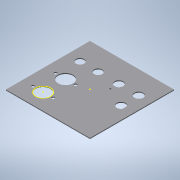
# Autodesk Inventor part: AmplifierPowerSupplyNew
Saved by Autodesk Inventor 2020 (Build 240168000, 168)
## iProperties
Created: 2013-08-12
Part Number: AmplifierPowerSupplyNew
Material: Generic
Document SubType Name: Modeling
Designer: laird
Density: 1 g/cm^3
Appearance: Default
Mass: 14.4778 g
Surface Area: 298.659 cm^2
Volume: 14.4778 cm^3
Author: laird
Title: Top plate
Autodesk Inventor part; units mm, degrees
ref_plane "YZ Plane" through (0, 0, 0) normal (1, 0, 0) x (0, 1, 0)
ref_plane "XZ Plane" through (0, 0, 0) normal (0, 1, 0) x (-1, 0, 0)
ref_plane "XY Plane" through (0, 0, 0) normal (0, 0, 1) x (1, 0, 0)
sketch "Sketch1" plane through (0, 0, 0) normal (0, 0, 1) x (1, 0, 0)
  line L0 (0, 46.5) -> (46.5, 46.5)
  line L1 (46.5, 46.5) -> (46.5, 0)
  line L2 (46.5, 0) -> (46.5, -46.5)
  line L3 (46.5, -46.5) -> (0, -46.5)
  line L4 (0, -46.5) -> (-46.5, -46.5)
  line L5 (-46.5, -46.5) -> (-46.5, 0)
  line L6 (-46.5, 0) -> (-46.5, 46.5)
  line L7 (-46.5, 46.5) -> (0, 46.5)
  point P0 (0, 0)
  dimension "d82" = 46.5
  dimension "d83" = 46.5
  dimension "d84" = 93
  dimension "d85" = 93
  constraints: 16 end point, 4 perpendicular, 4 point on line, 1 horizontal
  measures "d82" distance of L1.end L2.end
  measures "d83" distance of L3.end L4.end
  measures "d84" distance of L0.end L6.end
  measures "d85" distance of L2.end L0.end
extrude "Plate" add sketch "Sketch1" along normal blind 1
sketch "Sketch2" plane through (0, 0, 1) normal (0, 0, 1) x (1, 0, 0)
  circle A0 centre (-23.5, -28.5) radius 8.25
  circle A1 centre (-12.4, -28.5) radius 1.7
  circle A2 centre (-34.6, -28.5) radius 1.7
  line L0 (-46.5, 46.5) -> (-46.5, -46.5) projected
  line L1 (-46.5, -46.5) -> (46.5, -46.5) projected
  point P0 (0, 0)
  dimension "d6" = 16.5
  dimension "d8" = 3.4
  dimension "d29" = 11.1
  dimension "d30" = 11.1
  dimension "d93" = 23
  dimension "d94" = 18
  constraints: 3 centre point, 1 equal radius
  measures "d6" diameter of A0
  measures "d8" diameter of A2
  measures "d29" distance of A0.centre A1.centre
  measures "d30" distance of A0.centre A2.centre
  measures "d93" distance from line of L0 A0.centre
  measures "d94" distance from line of L1 A0.centre
extrude "DIN hole" cut sketch "Sketch2" against normal through all
pattern_linear "Rectangular Pattern1" count 2 spacing 25 along (0, 1, 0) of "DIN hole"
sketch "Sketch4" plane through (0, 0, 1) normal (0, 0, 1) x (1, 0, 0)
  circle A0 centre (-23.5, -28.5) radius 8.25 projected
  point P0 (0, 0)
sketch "Sketch5" plane through (0, 0, 1) normal (0, 0, 1) x (1, 0, 0)
  line L0 (46.5, 46.5) -> (-46.5, 46.5) projected
  line L1 (-46.5, 46.5) -> (-46.5, -46.5) projected
  circle A0 centre (-32.5, 21.5) radius 4.5
  point P0 (0, 0)
  dimension "d90" = 9
  dimension "d91" = 14
  dimension "d92" = 25
  constraints: 1 centre point
  measures "d90" diameter of A0
  measures "d91" distance from line of L1 A0.centre
  measures "d92" distance from line of L0 A0.centre
extrude "LED" cut sketch "Sketch5" along normal through all both and the other way through all
pattern_linear "Rectangular Pattern3" count 2 spacing 20 along (1, 0, 0) of "LED"
sketch "Sketch6" plane through (0, 0, 1) normal (0, 0, 1) x (1, 0, 0)
  circle A0 centre (32.5, 21.5) radius 4.85
  point P0 (-26.5, 37.5)
  point P1 (0, 0)
  dimension "d61" = 9.7
  constraints: 1 centre point
  measures "d61" diameter of A0
extrude "BNCs" cut sketch "Sketch6" along normal through all both and the other way through all
sketch "Sketch7" plane through (0, 0, 1) normal (0, 0, 1) x (1, 0, 0)
  circle A0 centre (32.5, 21.5) radius 4.85 projected
  circle A1 centre (10.5, 21.5) radius 4.75
  circle A2 centre (10.5, 12) radius 0.8
  point P0 (0, 0)
  dimension "d70" = 9.5
  dimension "d71" = 1.6
  dimension "d72" = 9.5
  dimension "d73" = 22
  constraints: 2 centre point, 1 vertical alignment
  measures "d70" diameter of A1
  measures "d71" diameter of A2
  measures "d72" distance of A2.centre A1.centre
  measures "d73" distance of A1.centre A0.centre
extrude "Extrusion9" cut sketch "Sketch7" against normal blind 1 contours A1 | A2
sketch "Sketch8" plane through (0, 0, 1) normal (0, 0, 1) x (1, 0, 0)
  arc A0 (36.5, 4.7427) -> (36.5, -0.7427) centre (32.5, 2) ccw
  line L0 (36.5, 2) -> (36.5, -0.7427)
  line L1 (36.5, 2) -> (36.5, 4.7427)
  point P0 (0, 0)
  constraints: 4 end point, 2 point on circle, 1 centre point, 1 point on line
extrude "Extrusion10" cut sketch "Sketch8" against normal blind 10
body "Solid1"
